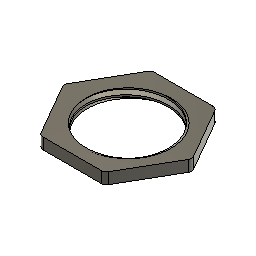
Nut_motor_coupling (Autodesk Fusion 360 design; units mm, degrees)
part number: 2025-04-25-16-47-41-473
Autodesk Fusion 360 part; units mm, degrees
sketch "Sketch1" plane through (0, 0, 0) normal (0, 1, 0) x (1, 0, 0)
  circle A0 centre (0, 0) radius 20
  line L0 (-14.4338, 25) -> (-28.8675, 0)
  line L1 (-28.8675, 0) -> (-14.4338, -25)
  line L2 (-14.4338, -25) -> (14.4338, -25)
  line L3 (14.4338, -25) -> (28.8675, 0)
  line L4 (28.8675, 0) -> (14.4338, 25)
  line L5 (14.4338, 25) -> (-14.4338, 25)
  dimension "d1" = 40
  constraint coincident A0.centre origin
  measures "d1" diameter of A0
extrude "Extrude1" add sketch "Sketch1" along normal blind 5
thread "Thread1" "ISO Metric profile 40.0 M40x3 6H" major diameter 40.349 minor diameter 37.0024 pitch 3 angle 60 modelled right hand crest width 0.8179 on face at (19.9751, 3.3333, 0.9969) crest through (18.5012, 0.75, 0)
fillet "Fillet1" radius 2.5 6 edges at (14.4338, 2.5, -25) (28.8675, 2.5, 0) (14.4338, 2.5, 25) (-14.4338, 2.5, 25) (-14.4338, 2.5, -25) (-28.8675, 2.5, 0)
